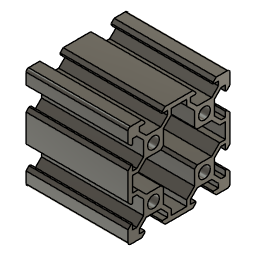
4040 V-Slot Forseti Cube (Autodesk Fusion 360 design; units mm, degrees)
Autodesk Fusion 360 part; units mm, degrees
sketch "Sketch1" plane through (0, 0, 0) normal (1, 0, 0) x (0, 1, 0)
  line L0 (20, 20) -> (-20, 20) construction
  line L1 (-20, 20) -> (-20, -20) construction
  line L2 (-20, -20) -> (20, -20) construction
  line L3 (20, -20) -> (20, 20) construction
  line L4 (20, 20) -> (-20, -20) construction
  line L5 (-20, 20) -> (20, -20) construction
  circle A0 centre (-10, 10) radius 2.3
  circle A1 centre (10, 10) radius 2.3
  circle A2 centre (-10, -10) radius 2.3
  circle A3 centre (10, -10) radius 2.3
  line L6 (18.2, 18.2) -> (-18.2, 18.2) construction
  line L7 (-18.2, 18.2) -> (-18.2, -18.2) construction
  line L8 (-18.2, -18.2) -> (18.2, -18.2) construction
  line L9 (18.2, -18.2) -> (18.2, 18.2) construction
  line L10 (-13.9, 12.8393) -> (-13.9, -12.8393) construction
  line L11 (-13.9, -13.9) -> (12.8393, -13.9) construction
  line L12 (13.9, -12.8393) -> (13.9, 12.8393) construction
  line L13 (10, 10) -> (-10, 10) construction
  line L14 (-10, 10) -> (-10, -10) construction
  line L15 (-10, -10) -> (10, -10) construction
  line L16 (10, -10) -> (10, 10) construction
  line L17 (10, 10) -> (-10, -10) construction
  line L18 (-10, 10) -> (10, -10) construction
  line L19 (6.1, 6.1) -> (-6.1, 6.1) construction
  line L20 (-6.1, 6.1) -> (-6.1, -6.1) construction
  line L21 (-6.1, -6.1) -> (6.1, -6.1) construction
  line L22 (6.1, -6.1) -> (6.1, 6.1) construction
  line L23 (-12.8393, 13.9) -> (-7.1607, 13.9)
  line L24 (-6.1, 12.8393) -> (-6.1, 6.1)
  line L25 (-6.1, 6.1) -> (-12.8393, 6.1)
  line L26 (-13.9, 6.1) -> (-13.9, 12.8393)
  line L27 (7.1607, 13.9) -> (12.8393, 13.9)
  line L28 (13.9, 12.8393) -> (13.9, 6.1)
  line L29 (13.9, 6.1) -> (6.1, 6.1)
  line L30 (6.1, 6.1) -> (6.1, 13.9)
  line L31 (-12.8393, -6.1) -> (-6.1, -6.1)
  line L32 (-6.1, -6.1) -> (-6.1, -12.8393)
  line L33 (-6.1, -13.9) -> (-13.9, -13.9)
  line L34 (-13.9, -12.8393) -> (-13.9, -6.1)
  line L35 (6.1, -6.1) -> (12.8393, -6.1)
  line L36 (13.9, -7.1607) -> (13.9, -12.8393)
  line L37 (12.8393, -13.9) -> (6.1, -13.9)
  line L38 (6.1, -12.8393) -> (6.1, -6.1)
  line L39 (-13.9, 12.8393) -> (-16.5607, 15.5)
  line L40 (-12.8393, 13.9) -> (-15.5, 16.5607)
  line L41 (-15.5, 16.5607) -> (-15.5, 18.2)
  line L42 (-16.5607, 15.5) -> (-18.2, 15.5)
  line L43 (-4.5, 18.2) -> (-4.5, 16.5607)
  line L44 (-18.2, 4.5) -> (-17.3803, 4.5)
  line L45 (-7.1607, 13.9) -> (-4.5, 16.5607)
  line L46 (-6.1, 12.8393) -> (-3, 15.9393)
  line L47 (-3, 15.9393) -> (-3, 18.2)
  line L48 (-15.5, 18.2) -> (-13.395, 18.2)
  line L49 (-6.605, 18.2) -> (-4.5, 18.2)
  line L50 (-20, 20) -> (-14.58, 20)
  line L51 (0, 20) -> (-5.42, 20)
  line L52 (-13.395, 18.2) -> (-13.395, 18.815)
  line L53 (-6.605, 18.2) -> (-6.605, 18.815)
  line L54 (-14.58, 20) -> (-13.395, 18.815)
  line L55 (-6.605, 18.815) -> (-5.42, 20)
  line L56 (-3, 18.2) -> (0, 18.2)
  line L57 (12.8393, 13.9) -> (-6.1, 13.9) construction
  line L58 (-7.1607, 13.9) -> (-13.9, 13.9) construction
  line L59 (-13.9, 13.9) -> (-13.9, 12.8393) construction
  line L60 (-6.1, 13.9) -> (-7.1607, 13.9) construction
  line L61 (-6.1, 13.9) -> (-6.1, 12.8393) construction
  line L62 (-20, 20) -> (-20, 14.58)
  line L63 (-18.2, 13.395) -> (-18.815, 13.395)
  line L64 (-18.2, 15.5) -> (-18.2, 13.395)
  line L65 (-16.5607, 15.5) -> (-18.2, 15.5)
  line L66 (-13.9, 12.8393) -> (-16.5607, 15.5)
  line L67 (-13.9, 12.8393) -> (-13.9, 7.1607)
  line L68 (-13.9, 7.1607) -> (-16.5607, 4.5)
  line L69 (-18.2, 4.5) -> (-16.5607, 4.5)
  line L70 (-18.2, 6.605) -> (-18.2, 4.5)
  line L71 (-18.2, 6.605) -> (-18.815, 6.605)
  line L72 (-18.815, 6.605) -> (-20, 5.42)
  line L73 (-20, 0) -> (-20, 5.42)
  line L74 (-20, 14.58) -> (-18.815, 13.395)
  line L75 (-12.8393, 6.1) -> (-15.9393, 3)
  line L76 (-15.9393, 3) -> (-18.2, 3)
  line L77 (18.2, 18.2) -> (18.2, -18.2) construction
  line L78 (18.2, -18.2) -> (-18.2, -18.2) construction
  line L79 (0, 0) -> (0, 6.1) construction
  line L80 (0, 0) -> (6.1, 0) construction
  line L81 (20, 20) -> (20, 14.58)
  line L82 (20, 14.58) -> (18.815, 13.395)
  line L83 (18.2, 13.395) -> (18.815, 13.395)
  line L84 (18.2, 15.5) -> (18.2, 13.395)
  line L85 (16.5607, 15.5) -> (18.2, 15.5)
  line L86 (13.9, 12.8393) -> (16.5607, 15.5)
  line L87 (13.9, 12.8393) -> (13.9, 7.1607)
  line L88 (18.2, 4.5) -> (16.5607, 4.5)
  line L89 (18.2, 6.605) -> (18.2, 4.5)
  line L90 (18.2, 6.605) -> (18.815, 6.605)
  line L91 (18.815, 6.605) -> (20, 5.42)
  line L92 (20, 0) -> (20, 5.42)
  line L93 (13.9, 7.1607) -> (16.5607, 4.5)
  line L94 (3, 18.2) -> (0, 18.2)
  line L95 (3, 15.9393) -> (3, 18.2)
  line L96 (6.1, 12.8393) -> (3, 15.9393)
  line L97 (6.1, 12.8393) -> (6.1, 6.1)
  line L98 (6.1, 6.1) -> (12.8393, 6.1)
  line L99 (15.9393, 3) -> (18.2, 3)
  line L100 (12.8393, 6.1) -> (15.9393, 3)
  line L101 (20, 20) -> (14.58, 20)
  line L102 (14.58, 20) -> (13.395, 18.815)
  line L103 (13.395, 18.2) -> (13.395, 18.815)
  line L104 (15.5, 18.2) -> (13.395, 18.2)
  line L105 (15.5, 16.5607) -> (15.5, 18.2)
  line L106 (12.8393, 13.9) -> (15.5, 16.5607)
  line L107 (7.1607, 13.9) -> (4.5, 16.5607)
  line L108 (4.5, 18.2) -> (4.5, 16.5607)
  line L109 (6.605, 18.2) -> (4.5, 18.2)
  line L110 (6.605, 18.2) -> (6.605, 18.815)
  line L111 (6.605, 18.815) -> (5.42, 20)
  line L112 (0, 20) -> (5.42, 20)
  line L113 (12.8393, 13.9) -> (7.1607, 13.9)
  line L114 (-20, -20) -> (-20, -14.58)
  line L115 (-20, -14.58) -> (-18.815, -13.395)
  line L116 (-18.2, -13.395) -> (-18.815, -13.395)
  line L117 (-18.2, -15.5) -> (-18.2, -13.395)
  line L118 (-16.5607, -15.5) -> (-18.2, -15.5)
  line L119 (-13.9, -12.8393) -> (-16.5607, -15.5)
  line L120 (-13.9, -12.8393) -> (-13.9, -7.1607)
  line L121 (-13.9, -7.1607) -> (-16.5607, -4.5)
  line L122 (-18.2, -4.5) -> (-16.5607, -4.5)
  line L123 (-18.2, -6.605) -> (-18.2, -4.5)
  line L124 (-18.2, -6.605) -> (-18.815, -6.605)
  line L125 (-18.815, -6.605) -> (-20, -5.42)
  line L126 (-20, 0) -> (-20, -5.42)
  line L127 (-3, -18.2) -> (0, -18.2)
  line L128 (-3, -15.9393) -> (-3, -18.2)
  line L129 (-6.1, -12.8393) -> (-3, -15.9393)
  line L130 (-6.1, -12.8393) -> (-6.1, -6.1)
  line L131 (-12.8393, -6.1) -> (-15.9393, -3)
  line L132 (-15.9393, -3) -> (-18.2, -3)
  line L133 (-6.1, -6.1) -> (-12.8393, -6.1)
  line L134 (-20, -20) -> (-14.58, -20)
  line L135 (-14.58, -20) -> (-13.395, -18.815)
  line L136 (-13.395, -18.2) -> (-13.395, -18.815)
  line L137 (-15.5, -18.2) -> (-13.395, -18.2)
  line L138 (-15.5, -16.5607) -> (-15.5, -18.2)
  line L139 (-12.8393, -13.9) -> (-15.5, -16.5607)
  line L140 (-12.8393, -13.9) -> (-7.1607, -13.9)
  line L141 (-4.5, -18.2) -> (-4.5, -16.5607)
  line L142 (-6.605, -18.2) -> (-4.5, -18.2)
  line L143 (-6.605, -18.2) -> (-6.605, -18.815)
  line L144 (-6.605, -18.815) -> (-5.42, -20)
  line L145 (0, -20) -> (-5.42, -20)
  line L146 (-7.1607, -13.9) -> (-4.5, -16.5607)
  line L147 (20, -20) -> (14.58, -20)
  line L148 (14.58, -20) -> (13.395, -18.815)
  line L149 (13.395, -18.2) -> (13.395, -18.815)
  line L150 (15.5, -18.2) -> (13.395, -18.2)
  line L151 (15.5, -16.5607) -> (15.5, -18.2)
  line L152 (12.8393, -13.9) -> (15.5, -16.5607)
  line L153 (12.8393, -13.9) -> (7.1607, -13.9)
  line L154 (4.5, -18.2) -> (4.5, -16.5607)
  line L155 (6.605, -18.2) -> (4.5, -18.2)
  line L156 (6.605, -18.2) -> (6.605, -18.815)
  line L157 (6.605, -18.815) -> (5.42, -20)
  line L158 (0, -20) -> (5.42, -20)
  line L159 (7.1607, -13.9) -> (4.5, -16.5607)
  line L160 (3, -18.2) -> (0, -18.2)
  line L161 (3, -15.9393) -> (3, -18.2)
  line L162 (6.1, -12.8393) -> (3, -15.9393)
  line L163 (6.1, -6.1) -> (12.8393, -6.1)
  line L164 (12.8393, -6.1) -> (15.9393, -3)
  line L165 (15.9393, -3) -> (18.2, -3)
  line L166 (6.1, -12.8393) -> (6.1, -6.1)
  line L167 (20, -20) -> (20, -14.58)
  line L168 (20, -14.58) -> (18.815, -13.395)
  line L169 (18.2, -13.395) -> (18.815, -13.395)
  line L170 (18.2, -15.5) -> (18.2, -13.395)
  line L171 (16.5607, -15.5) -> (18.2, -15.5)
  line L172 (13.9, -12.8393) -> (16.5607, -15.5)
  line L173 (13.9, -12.8393) -> (13.9, -7.1607)
  line L174 (18.2, -4.5) -> (16.5607, -4.5)
  line L175 (18.2, -6.605) -> (18.2, -4.5)
  line L176 (18.2, -6.605) -> (18.815, -6.605)
  line L177 (18.815, -6.605) -> (20, -5.42)
  line L178 (20, 0) -> (20, -5.42)
  line L179 (-18.2, 3) -> (-18.2, -3) construction
  line L180 (-18.2, 3) -> (-18.2, -3)
  line L181 (18.2, 3) -> (18.2, -3)
  line L182 (13.9, -7.1607) -> (16.5607, -4.5)
  point P0 (-10, 10)
  dimension "d1" = 40
  dimension "d2" = 40
  dimension "d3" = 10
  dimension "d4" = 4.6
  dimension "d7" = 20
  dimension "d8" = -20
  dimension "d9" = -1.8
  dimension "d14" = -3.9
  dimension "d22" = 1.5
  dimension "d23" = 11
  dimension "d24" = 11
  dimension "d25" = 1.5
  dimension "d26" = 135
  dimension "d27" = 1.5
  dimension "d28" = 6.79
  dimension "d29" = 9.16
  dimension "d30" = 135
  dimension "d31" = 135
  constraint horizontal L0
  constraint perpendicular L0 L1
  constraint parallel L0 L2
  constraint parallel L1 L3
  constraint coincident L4 L79.start
  constraint coincident L5 L79.start
  constraint coincident L79.start L80.start
  constraint coincident L5 P0
  constraint coincident P0 A0.centre
  constraint horizontal L13
  constraint perpendicular L13 L14
  constraint parallel L13 L15
  constraint parallel L14 L16
  constraint coincident L17 L79.start
  constraint coincident L18 L79.start
  constraint coincident A1.centre L13.start
  constraint horizontal L23
  constraint vertical L24
  constraint horizontal L25
  constraint vertical L26
  constraint parallel L5 L39
  constraint coincident L23.start L57
  constraint parallel L39 L40
  constraint symmetric L5 L39 L40
  constraint coincident L6 L41.end
  constraint perpendicular L6 L41
  constraint coincident L7 L42.end
  constraint perpendicular L7 L42
  constraint coincident L6 L43.start
  constraint vertical L43
  constraint symmetric L14 L41 L43
  constraint coincident L7 L44.start
  constraint perpendicular L7 L44
  constraint parallel L45 L46
  constraint horizontal L40.end L43.end
  constraint coincident L6 L47.end
  constraint perpendicular L6 L47
  constraint coincident L6 L48.end
  constraint coincident L6 L49.start
  constraint coincident L0 L50.end
  constraint midpoint L0 L51.start
  constraint coincident L0 L51.end
  constraint symmetric L14 L50.end L51.end
  constraint symmetric L14 L48.end L49.start
  constraint perpendicular L6 L52
  constraint perpendicular L49 L53
  constraint midpoint L6 L56.end
  constraint collinear L57 L58
  constraint perpendicular L58 L59
  constraint perpendicular L60 L61
  constraint symmetric L0.end L5 L1.start
  constraint symmetric L5 L6.start L7.end
  constraint symmetric L5 L7.end L6.start
  constraint symmetric L5 L8.end L9.start
  constraint symmetric L5 L23.start L10.start
  constraint symmetric L5 L40.end L39.end
  constraint symmetric L5 L41.end L42.end
  constraint symmetric L5 L43.start L44.start
  constraint symmetric L5 L43.end L68.end
  constraint symmetric L5 L23.end L67.end
  constraint symmetric L5 L24.start L25.end
  constraint symmetric L5 L46.end L75.end
  constraint symmetric L5 L47.end L76.end
  constraint symmetric L5 L48.end L63.start
  constraint symmetric L5 L49.start L70.start
  constraint symmetric L5 L50.end L62.end
  constraint symmetric L5 L51.start L73.start
  constraint symmetric L5 L51.end L72.end
  constraint symmetric L5 L52.end L63.end
  constraint symmetric L5 L53.end L71.end
  constraint midpoint L19 L79.end
  constraint midpoint L22 L80.end
  constraint symmetric L0.end L79 L0.start
  constraint symmetric L19.end L79 L19.start
  constraint symmetric L23.start L79 L27.end
  constraint symmetric L40.end L79 L105.start
  constraint symmetric L41.end L79 L104.start
  constraint symmetric L43.start L79 L108.start
  constraint symmetric L43.end L79 L107.end
  constraint symmetric L23.end L79 L27.start
  constraint symmetric L24.start L79 L96.start
  constraint symmetric L46.end L79 L95.start
  constraint symmetric L47.end L79 L94.start
  constraint symmetric L48.end L79 L103.start
  constraint symmetric L49.start L79 L109.start
  constraint symmetric L50.end L79 L101.end
  constraint symmetric L51.start L79 L112.start
  constraint symmetric L51.end L79 L111.end
  constraint symmetric L52.end L79 L102.end
  constraint symmetric L53.end L79 L110.end
  constraint symmetric L56.end L79 L94.end
  constraint symmetric L62.end L79 L81.end
  constraint symmetric L63.start L79 L83.start
  constraint symmetric L63.end L79 L82.end
  constraint symmetric L42.end L79 L84.start
  constraint symmetric L39.end L79 L85.start
  constraint symmetric L10.start L79 L12.end
  constraint symmetric L67.end L79 L87.end
  constraint symmetric L68.end L79 L88.end
  constraint symmetric L44.start L79 L88.start
  constraint symmetric L70.start L79 L89.start
  constraint symmetric L71.end L79 L90.end
  constraint symmetric L72.end L79 L91.end
  constraint symmetric L73.start L79 L92.start
  constraint symmetric L25.end L79 L98.end
  constraint symmetric L75.end L79 L99.start
  constraint symmetric L76.end L79 L99.end
  constraint symmetric L0.end L80 L1.end
  constraint symmetric L19.end L80 L20.end
  constraint symmetric L23.start L80 L139.start
  constraint symmetric L40.end L80 L138.start
  constraint symmetric L41.end L80 L137.start
  constraint symmetric L43.start L80 L141.start
  constraint symmetric L43.end L80 L141.end
  constraint symmetric L23.end L80 L140.end
  constraint symmetric L24.start L80 L32.end
  constraint symmetric L46.end L80 L128.start
  constraint symmetric L47.end L80 L127.start
  constraint symmetric L48.end L80 L136.start
  constraint symmetric L49.start L80 L142.start
  constraint symmetric L50.end L80 L134.end
  constraint symmetric L51.start L80 L145.start
  constraint symmetric L51.end L80 L144.end
  constraint symmetric L52.end L80 L135.end
  constraint symmetric L53.end L80 L143.end
  constraint symmetric L56.end L80 L127.end
  constraint symmetric L62.end L80 L114.end
  constraint symmetric L63.start L80 L116.start
  constraint symmetric L63.end L80 L115.end
  constraint symmetric L42.end L80 L117.start
  constraint symmetric L39.end L80 L118.start
  constraint symmetric L10.start L80 L10.end
  constraint symmetric L67.end L80 L120.end
  constraint symmetric L68.end L80 L121.end
  constraint symmetric L44.start L80 L122.start
  constraint symmetric L70.start L80 L123.start
  constraint symmetric L71.end L80 L124.end
  constraint symmetric L72.end L80 L125.end
  constraint symmetric L73.start L80 L126.start
  constraint symmetric L25.end L80 L31.start
  constraint symmetric L75.end L80 L131.end
  constraint symmetric L76.end L80 L132.end
  constraint symmetric L80 L0.start L2.end
  constraint symmetric L80 L81.end L167.end
  constraint symmetric L80 L82.end L168.end
  constraint symmetric L80 L83.start L169.start
  constraint symmetric L80 L84.start L170.start
  constraint symmetric L80 L85.start L171.start
  constraint symmetric L80 L12.end L12.start
  constraint symmetric L80 L87.end L36.start
  constraint symmetric L80 L88.start L174.start
  constraint symmetric L80 L88.end L174.end
  constraint symmetric L80 L89.start L175.start
  constraint symmetric L80 L90.end L176.end
  constraint symmetric L80 L91.end L177.end
  constraint symmetric L80 L92.start L178.start
  constraint symmetric L80 L94.start L160.start
  constraint symmetric L80 L56.end L127.end
  constraint symmetric L80 L95.start L161.start
  constraint symmetric L80 L96.start L38.start
  constraint symmetric L80 L19.start L21.end
  constraint symmetric L80 L98.end L35.end
  constraint symmetric L80 L99.start L164.end
  constraint symmetric L80 L99.end L165.end
  constraint symmetric L80 L101.end L147.end
  constraint symmetric L80 L102.end L148.end
  constraint symmetric L80 L103.start L149.start
  constraint symmetric L80 L104.start L150.start
  constraint symmetric L80 L105.start L151.start
  constraint symmetric L80 L27.end L11.end
  constraint symmetric L80 L27.start L153.end
  constraint symmetric L80 L107.end L154.end
  constraint symmetric L80 L108.start L154.start
  constraint symmetric L80 L109.start L155.start
  constraint symmetric L80 L110.end L156.end
  constraint symmetric L80 L111.end L157.end
  constraint symmetric L80 L51.start L145.start
  constraint midpoint L44.end L69
  measures "d1" distance of L1.end L2.end
  measures "d2" distance of L0.end L1.end
  measures "d3" distance of L0 P0
  measures "d4" diameter of A0
  measures "d22" distance of L39 L40
  measures "d23" distance of L41 L43
  measures "d24" distance of L42 L44
  measures "d25" distance of L45 L46
  measures "d26" angle of L23 L45
  measures "d27" distance of L43 L47
  measures "d28" distance of L48.end L49.start
  measures "d29" distance of L50.end L51.end
  measures "d30" angle of L53 L55
  measures "d31" angle of L52 L54
extrude "Extrude1" add sketch "Sketch1" along normal blind 40
chamfer "Chamfer2" distance 1 angle 45 4 edges at (20, 6.1, 6.1) (20, -6.1, 6.1) (20, -6.1, -6.1) (20, 6.1, -6.1)
fillet "Fillet1" radius 1 4 edges at (20, 20, -20) (20, -20, -20) (20, -20, 20) (20, 20, 20)
named bodies: "4040 V-Slot Forseti"
